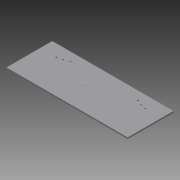
# Autodesk Inventor part: Camera Rig Base
Saved by Autodesk Inventor 2013 (Build 170138000, 138)
## iProperties
Created: 2013-03-16
Part Number: Camera Rig Base
Material: Generic
Document SubType Name: Modeling
Designer: tyler.camp
Density: 1 g/cm^3
Author: tyler.camp
Autodesk Inventor part; units mm, degrees
ref_plane "YZ Plane" through (0, 0, 0) normal (1, 0, 0) x (0, 1, 0)
ref_plane "XZ Plane" through (0, 0, 0) normal (0, 1, 0) x (-1, 0, 0)
ref_plane "XY Plane" through (0, 0, 0) normal (0, 0, 1) x (1, 0, 0)
sketch "Sketch1" plane through (0, 0, 0) normal (0, 1, 0) x (-1, 0, 0)
  line L0 (-225, 85) -> (225, 85)
  line L1 (225, 85) -> (225, -85)
  line L2 (225, -85) -> (-225, -85)
  line L3 (-225, -85) -> (-225, 85)
  point P0 (0, 0)
  dimension "d0" = 450
  dimension "d2" = 170
  dimension "d3" = 225
  dimension "d4" = 85
  constraints: 8 end point, 2 parallel, 1 horizontal, 1 perpendicular
  measures "d0" distance of L0.start L0.end
  measures "d2" distance of L2.end L0.start
  measures "d3" distance from line of point (0, 0) L3
  measures "d4" distance from line of point (0, 0) L0
extrude "Extrusion1" add sketch "Sketch1" along normal blind 5
sketch "Sketch2" plane through (0, 5, 0) normal (0, 1, 0) x (1, 0, 0)
  line L0 (-225, -85) -> (225, -85) projected
  line L1 (225, -85) -> (225, 85) projected
  line L2 (-225, 85) -> (-225, -85) projected
  circle A0 centre (-165, 40) radius 2.5
  circle A1 centre (-145, 45) radius 2.5
  circle A2 centre (-125, 52.5) radius 2.5
  circle A3 centre (125, 52.5) radius 2.5
  circle A4 centre (145, 45) radius 2.5
  circle A5 centre (165, 40) radius 2.5
  circle A6 centre (-20, -5) radius 1.25
  circle A7 centre (-20, 5) radius 1.25
  circle A8 centre (20, -5) radius 1.25
  circle A9 centre (20, 5) radius 1.25
  point P0 (0, 0)
  dimension "d7" = 137.5
  dimension "d8" = 130
  dimension "d9" = 125
  dimension "d10" = 60
  dimension "d11" = 80
  dimension "d12" = 100
  dimension "d13" = 100
  dimension "d14" = 80
  dimension "d15" = 60
  dimension "d16" = 125
  dimension "d17" = 130
  dimension "d18" = 137.5
  dimension "d19" = 20
  dimension "d20" = 20
  dimension "d21" = 20
  dimension "d22" = 20
  dimension "d23" = 80
  dimension "d24" = 80
  dimension "d26" = 10
  dimension "d27" = 10
  dimension "d28" = 5
  dimension "d29" = 5
  dimension "d30" = 5
  dimension "d31" = 5
  dimension "d32" = 5
  dimension "d33" = 5
  dimension "d34" = 2.5
  dimension "d35" = 2.5
  dimension "d36" = 2.5
  dimension "d37" = 2.5
  constraints: 10 centre point, 10 coincident
  measures "d7" distance from line of L0 point (-125, 52.5)
  measures "d8" distance from line of L0 point (-145, 45)
  measures "d9" distance from line of L0 point (-165, 40)
  measures "d10" distance from line of L2 point (-165, 40)
  measures "d11" distance from line of L2 point (-145, 45)
  measures "d12" distance from line of L2 point (-125, 52.5)
  measures "d13" distance from line of L1 point (125, 52.5)
  measures "d14" distance from line of L1 point (145, 45)
  measures "d15" distance from line of L1 point (165, 40)
  measures "d16" distance from line of L0 point (165, 40)
  measures "d17" distance from line of L0 point (145, 45)
  measures "d18" distance from line of L0 point (125, 52.5)
  measures "d19" horizontal distance of point (0, 0) point (-20, -5)
  measures "d20" horizontal distance of point (0, 0) point (-20, 5)
  measures "d21" horizontal distance of point (0, 0) point (20, 5)
  measures "d22" horizontal distance of point (0, 0) point (20, -5)
  measures "d23" distance from line of L0 point (-20, -5)
  measures "d24" distance from line of L0 point (20, -5)
  measures "d26" distance of point (20, 5) point (20, -5)
  measures "d27" distance of point (-20, -5) point (-20, 5)
  measures "d28" diameter of A0
  measures "d29" diameter of A1
  measures "d30" diameter of A2
  measures "d31" diameter of A3
  measures "d32" diameter of A4
  measures "d33" diameter of A5
  measures "d34" diameter of A6
  measures "d35" diameter of A7
  measures "d36" diameter of A8
  measures "d37" diameter of A9
extrude "Extrusion2" cut sketch "Sketch2" against normal through all
equation "\"d3\" = 0.5 * d0"
equation "\"d4\" = 0.5 * d2"
body "Solid1"
